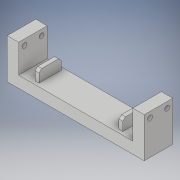
# Autodesk Inventor part: 000.201 - Балка несущая
Saved by Autodesk Inventor 2019 (Build 230136000, 136)
## iProperties
Created: 2020-06-06
Part Number: 000.201 - Балка несущая
Material: Типовые
Document SubType Name: Modeling
Designer: Петров Иван
Density: 1 g/cm^3
Appearance: По умолчанию
Author: Петров Иван
Autodesk Inventor part; units mm, degrees
ref_plane "YZ Plane" through (0, 0, 0) normal (1, 0, 0) x (0, 1, 0)
ref_plane "XZ Plane" through (0, 0, 0) normal (0, 1, 0) x (-1, 0, 0)
ref_plane "XY Plane" through (0, 0, 0) normal (0, 0, 1) x (1, 0, 0)
sketch "Эскиз1" plane through (0, 0, 0) normal (0, 1, 0) x (-1, 0, 0)
  line L0 (50, 15.4) -> (40.5, 15.4)
  line L1 (50, 15.4) -> (-50, 15.4)
  line L2 (-50, -9.6) -> (-50, 15.4)
  line L3 (50, -9.6) -> (40.5, -9.6)
  line L4 (50, -9.6) -> (-50, -9.6)
  line L5 (50, 15.4) -> (-50, 15.4)
  line L6 (-50, 15.4) -> (-50, -9.6)
  line L7 (-50, -9.6) -> (50, -9.6)
  line L8 (50, -9.6) -> (50, 15.4)
  line L9 (38.4, 12.5) -> (38.4, -6.7)
  line L10 (38.4, 12.5) -> (35, 12.5)
  line L11 (35, 12.5) -> (35, -6.7)
  line L12 (35, -6.7) -> (38.4, -6.7)
  line L13 (38.4, -6.7) -> (38.4, 12.5)
  line L14 (-35, -9.6) -> (-35, 15.4)
  line L15 (-35, -9.6) -> (-38.4, -9.6)
  line L16 (-35, 15.4) -> (-38.4, 15.4)
  line L17 (-38.4, 15.4) -> (-38.4, -9.6)
  line L18 (-38.4, -9.6) -> (-35, -9.6)
  line L19 (-35, -9.6) -> (-35, 15.4)
  line L20 (50, 15.4) -> (60, 15.4)
  line L21 (60, 15.4) -> (60, -9.6)
  line L22 (60, -9.6) -> (50, -9.6)
  line L23 (50, -9.6) -> (50, 15.4)
  line L24 (-50, 15.4) -> (-60, 15.4)
  line L25 (-60, 15.4) -> (-60, -9.6)
  line L26 (-60, -9.6) -> (-50, -9.6)
  line L27 (-50, -9.6) -> (-50, 15.4)
  line L28 (-35, -6.7) -> (-38.4, -6.7)
  line L29 (-35, 12.5) -> (-38.4, 12.5)
  point P0 (0, 0)
  point P1 (0, 0)
  point P2 (50, 15.4)
  dimension "d10" = 25
  dimension "d1" = 10
  dimension "d2" = 10
  dimension "d9" = 25
  dimension "d11" = 2.9
  dimension "d12" = 25
  dimension "d13" = 2.9
  dimension "d15" = 2.9
  constraints: 56 end point, 10 parallel, 7 perpendicular, 7 point on line, 6 horizontal, 7 other
  measures "d1" distance of L21.end L22.end
  measures "d2" distance of L26.end L25.end
  measures "d9" distance of L20.end L21.end
  measures "d12" distance of L24.end L25.end
extrude "Выдавливание1" add sketch "Эскиз1" along normal blind 10 contours L8 L3 L4 L14 L1 L0 | L20 L21 L22 L8 | L14 L29 L17 L1 | L17 L4 L2 L1 | L14 L28 L17 L29 | L4 L17 L28 L14 | L2 L26 L25 L24 | L9 L12 L11 L10
sketch "Эскиз2" plane through (0, 10, 0) normal (0, 1, 0) x (1, 0, 0)
  line L0 (-60, 9.6) -> (-60, -15.4) projected
  line L1 (60, 9.6) -> (-60, 9.6) projected
  line L2 (-60, -15.4) -> (60, -15.4)
  line L3 (60, -15.4) -> (60, 9.6)
  line L4 (60, 9.6) -> (-60, 9.6)
  line L5 (-60, 9.6) -> (-60, -15.4)
  line L6 (60, -15.4) -> (60, 9.6) projected
  line L7 (60, -15.4) -> (50, -15.4)
  line L8 (50, -15.4) -> (50, 9.6)
  line L9 (50, 9.6) -> (60, 9.6)
  line L10 (60, 9.6) -> (60, -15.4)
  line L11 (-60, -15.4) -> (60, -15.4) projected
  line L12 (-60, -15.4) -> (-50, -15.4)
  line L13 (-50, -15.4) -> (-50, 9.6)
  line L14 (-50, 9.6) -> (-60, 9.6)
  line L15 (-60, 9.6) -> (-60, -15.4)
  dimension "d16" = 10
  dimension "d17" = 10
  constraints: 24 end point, 6 parallel, 3 horizontal, 3 perpendicular, 2 point on line
  measures "d16" distance of L8.end L9.end
  measures "d17" distance of L14.end L13.end
extrude "Выдавливание2" add sketch "Эскиз2" along normal blind 25 contours L1 L13 L2 L0 | L1 L3 L2 L8
sketch "Эскиз3" plane through (60, 0, 15.4) normal (1, 0, 0) x (0, 0, -1)
  line L0 (0, 25) -> (0, 35)
  line L1 (0, 30) -> (25, 30)
  line L2 (25, 25) -> (25, 35)
  circle A0 centre (5, 30) radius 2.1
  circle A1 centre (20, 30) radius 2.1
  line L3 (0, 35) -> (25, 35) projected
  point P0 (15.4, 0)
  point P1 (50, 0)
  dimension "d18" = 4.2
  dimension "d19" = 4.2
  dimension "d20" = 5
  dimension "d21" = 5
  constraints: 6 end point, 2 centre point, 2 midpoint, 2 point on line
  measures "d18" diameter of A0
  measures "d19" diameter of A1
  measures "d20" distance from line of L2 A1.centre
  measures "d21" distance from line of L0 A0.centre
extrude "Выдавливание3" cut sketch "Эскиз3" against normal blind 127.5 contours A0 L1 | L1 A0 | A1 L1 | L1 A1
sketch "Эскиз4" plane through (0, 10, 0) normal (0, 1, 0) x (1, 0, 0)
  line L0 (50, 9.6) -> (40.5, 9.6)
  line L1 (50, 9.6) -> (-50, 9.6)
  line L2 (-50, -15.4) -> (-50, 9.6)
  line L3 (50, -15.4) -> (40.5, -15.4)
  line L4 (50, -15.4) -> (-50, -15.4)
  line L5 (50, 9.6) -> (-50, 9.6)
  line L6 (-50, 9.6) -> (-50, -15.4)
  line L7 (-50, -15.4) -> (50, -15.4)
  line L8 (50, -15.4) -> (50, 9.6)
  line L9 (38.4, 6.7) -> (38.4, -12.5)
  line L10 (38.4, 6.7) -> (35, 6.7)
  line L11 (35, 6.7) -> (35, -12.5)
  line L12 (35, -12.5) -> (38.4, -12.5)
  line L13 (38.4, -12.5) -> (38.4, 6.7)
  line L14 (-35, -15.4) -> (-35, 9.6)
  line L15 (-35, -15.4) -> (-38.4, -15.4)
  line L16 (-35, 9.6) -> (-38.4, 9.6)
  line L17 (-38.4, 9.6) -> (-38.4, -15.4)
  line L18 (-38.4, -15.4) -> (-35, -15.4)
  line L19 (-35, -15.4) -> (-35, 9.6)
  line L20 (50, 9.6) -> (60, 9.6)
  line L21 (60, 9.6) -> (60, -15.4)
  line L22 (60, -15.4) -> (50, -15.4)
  line L23 (50, -15.4) -> (50, 9.6)
  line L24 (-50, 9.6) -> (-60, 9.6)
  line L25 (-60, 9.6) -> (-60, -15.4)
  line L26 (-60, -15.4) -> (-50, -15.4)
  line L27 (-50, -15.4) -> (-50, 9.6)
  line L28 (-35, -12.5) -> (-38.4, -12.5)
  line L29 (-35, 6.7) -> (-38.4, 6.7)
  point P0 (0, 0)
  point P1 (0, 0)
  point P2 (0, 0)
  point P3 (50, 9.6)
  dimension "d27" = 25
  dimension "d24" = 10
  dimension "d25" = 10
  dimension "d26" = 25
  dimension "d28" = 2.9
  dimension "d29" = 25
  dimension "d30" = 2.9
  dimension "d31" = 2.9
  constraints: 56 end point, 10 parallel, 7 perpendicular, 7 point on line, 6 horizontal, 7 other
  measures "d24" distance of L21.end L22.end
  measures "d25" distance of L26.end L25.end
  measures "d26" distance of L20.end L21.end
  measures "d29" distance of L24.end L25.end
extrude "Выдавливание4" add sketch "Эскиз4" along normal blind 10 contours L14 L28 L17 L29 | L9 L12 L11 L10
chamfer "Фаска1" distance 2.25 angle 45 4 edges at (-36.7, 20, 12.5) (-36.7, 20, -6.7) (36.7, 20, 12.5) (36.7, 20, -6.7)
equation "\"d19\" = d18"
equation "\"d20\" = d21"
